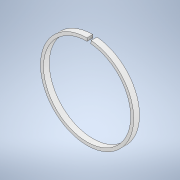
# Autodesk Inventor part: 4002_Bias_Coil_Holder_Tube_Mount_Layer3_MPSv2_v2
Saved by Autodesk Inventor 2021 (Build 250183000, 183)
## iProperties
Created: 2021-02-18
Part Number: 4002_Bias_Coil_Holder_Tube_Mount_Layer3_MPSv2_v2
Material: ABS Plastic
Document SubType Name: Modeling
Designer: Barksdale
Density: 1.06 g/cm^3
Appearance: Smooth - White
Author: Barksdale
Autodesk Inventor part; units mm, degrees
ref_plane "YZ Plane" through (0, 0, 0) normal (1, 0, 0) x (0, 1, 0)
ref_plane "XZ Plane" through (0, 0, 0) normal (0, 1, 0) x (-1, 0, 0)
ref_plane "XY Plane" through (0, 0, 0) normal (0, 0, 1) x (1, 0, 0)
sketch "Sketch1" plane through (0, 0, 0) normal (0, 0, 1) x (1, 0, 0)
  circle A0 centre (0, 0) radius 48.129
  circle A1 centre (0, 0) radius 45.0088
  dimension "d0" = 96.258
  dimension "d1" = 90.0176
  constraints: 2 centre point, 2 coincident
  measures "d0" diameter of A0
  measures "d1" diameter of A1
extrude "Extrusion1" add sketch "Sketch1" along normal blind 6
sketch "Sketch2" plane through (0, 0, 6) normal (0, 0, 1) x (1, 0, 0)
  line L0 (0, 0) -> (0, 63.8312)
  line L1 (0, 0) -> (5.4044, 61.7725)
  line L2 (0, 0) -> (62.0085, 0) construction
  line L3 (5.4044, 61.7725) -> (1.0128, 63.4454)
  line L4 (1.0128, 63.4454) -> (0, 63.8312)
  dimension "d4" = 85
  constraints: 10 end point, 1 collinear, 1 equal length, 1 horizontal, 1 vertical
  measures "d4" angle of L2 L1
extrude "Extrusion2" cut sketch "Sketch2" against normal blind 10
body "Solid1"
